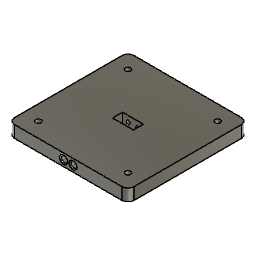
a_easy_one v3 (Autodesk Fusion 360 design; units mm, degrees)
Autodesk Fusion 360 part; units mm, degrees
sketch "Sketch1" plane through (0, 0, 0) normal (0, 0, 1) x (1, 0, 0)
  line L0 (0, 0) -> (100, 0)
  line L1 (100, 0) -> (100, 100)
  line L2 (100, 100) -> (0, 100)
  line L3 (0, 100) -> (0, 0)
  line L4 (12.5, 87.5) -> (87.5, 87.5) construction
  line L5 (87.5, 87.5) -> (87.5, 12.5) construction
  line L6 (87.5, 12.5) -> (12.5, 12.5) construction
  line L7 (12.5, 12.5) -> (12.5, 87.5) construction
  line L8 (87.5, 50) -> (12.5, 50) construction
  line L9 (50, 87.5) -> (50, 12.5) construction
  circle A0 centre (12.5, 87.5) radius 2.25
  circle A1 centre (87.5, 87.5) radius 2.25
  circle A2 centre (12.5, 12.5) radius 2.25
  circle A3 centre (87.5, 12.5) radius 2.25
  line L10 (41.3, 45.8) -> (58.7, 45.8)
  line L11 (58.7, 45.8) -> (58.7, 54.2)
  line L12 (58.7, 54.2) -> (41.3, 54.2)
  line L13 (41.3, 54.2) -> (41.3, 45.8)
  dimension "d1" = 100
  dimension "d3" = 75
  dimension "d4" = 4.5
  dimension "d5" = 17.4
  dimension "d6" = 8.4
  constraint horizontal L0
  constraint vertical L1
  constraint horizontal L2
  constraint vertical L3
  constraint coincident L0.start L3.end
  constraint equal L0 L3
  constraint horizontal L4
  constraint vertical L5
  constraint horizontal L6
  constraint vertical L7
  constraint equal L4 L7
  constraint midpoint L5 L8.start
  constraint midpoint L7 L8.end
  constraint midpoint L4 L9.start
  constraint midpoint L6 L9.end
  constraint symmetric L1 L3 L9
  constraint symmetric L0 L2 L8
  constraint coincident L4.start L7.end
  constraint coincident L4.end L5.start
  constraint coincident L6.end L7.start
  constraint coincident L5.end L6.start
  constraint equal A0 A1
  constraint equal A1 A3
  constraint equal A2 A3
  constraint horizontal L10
  constraint vertical L11
  constraint horizontal L12
  constraint vertical L13
  constraint symmetric L8 L10 L12
  constraint symmetric L9 L11 L13
  measures "d1" distance of L0.start L0.end
  measures "d3" distance of L4.start L6.end
  measures "d4" diameter of A2
  measures "d5" distance of L10.start L10.end
  measures "d6" distance of L10.end L11.end
extrude "Extrude1" add sketch "Sketch1" along normal blind 10
sketch "Sketch2" plane through (0, 100, 0) normal (0, 1, 0) x (-1, 0, 0)
  line L0 (-100, 0) -> (0, 0)
  line L1 (0, 0) -> (0, 10)
  line L2 (0, 10) -> (-100, 10)
  line L3 (-100, 10) -> (-100, 0)
  circle A0 centre (-54, 5) radius 1.65
  circle A1 centre (-46, 5) radius 1.65
  line L4 (-50, 10) -> (-50, 0) construction
  line L5 (-54, 5) -> (-46, 5) construction
  dimension "d11" = 8
  dimension "d14" = 3.3
  constraint midpoint L2 L4.start
  constraint midpoint L0 L4.end
  constraint coincident A0.centre L5.start
  constraint coincident A1.centre L5.end
  constraint parallel L0 L5
  constraint symmetric L0 L2 L5
  constraint symmetric A0 A1 L4
  measures "d11" distance of A0.centre A1.centre
  measures "d14" diameter of A1
extrude "Extrude2" cut sketch "Sketch2" against normal up to surface (100 mm away) contours A0 | A1
sketch "Sketch3" plane through (0, 100, 0) normal (0, 1, 0) x (-1, 0, 0)
  circle A0 centre (-54, 5) radius 1.65
  circle A1 centre (-46, 5) radius 1.65
  line L0 (-100, 0) -> (0, 0)
  line L1 (0, 0) -> (0, 10)
  line L2 (0, 10) -> (-100, 10)
  line L3 (-100, 10) -> (-100, 0)
  circle A2 centre (-54, 5) radius 2.55
  circle A3 centre (-46, 5) radius 2.55
  dimension "d15" = 5.1
  constraint concentric A0 A2
  constraint concentric A1 A3
  constraint equal A2 A3
  measures "d15" diameter of A2
extrude "Extrude3" cut sketch "Sketch3" against normal blind 8 contours A2 | A3
sketch "Sketch4" plane through (0, 0, 0) normal (0, -1, 0) x (1, 0, 0)
  circle A0 centre (54, 5) radius 1.65
  circle A1 centre (46, 5) radius 1.65
  line L0 (0, 0) -> (100, 0)
  line L1 (100, 0) -> (100, 10)
  line L2 (100, 10) -> (0, 10)
  line L3 (0, 10) -> (0, 0)
  circle A2 centre (46, 5) radius 2.55
  circle A3 centre (54, 5) radius 2.55
  dimension "d18" = 5.1
  constraint concentric A1 A2
  constraint concentric A0 A3
  constraint equal A2 A3
  measures "d18" diameter of A2
extrude "Extrude4" cut sketch "Sketch4" against normal blind 8 contours A2 | A3
fillet "Fillet1" radius 0.8 4 edges at (48.3774, 100, 5.9221) (56.3774, 100, 5.9221) (51.6226, 0, 5.9221) (43.6226, 0, 5.9221)
fillet "Fillet3" radius 5 4 edges at (100, 0, 5) (0, 0, 5) (100, 100, 5) (0, 100, 5)
